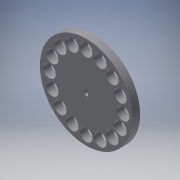
# Autodesk Inventor part: feeder_ring
Saved by Autodesk Inventor 2019 (Build 230136000, 136)
## iProperties
Created: 2018-11-14
Part Number: feeder_ring
Material: Generic
Document SubType Name: Modeling
Designer: chill
Density: 1 g/cm^3
Appearance: Default
Author: chill
Autodesk Inventor part; units mm, degrees
ref_plane "YZ Plane" through (0, 0, 0) normal (1, 0, 0) x (0, 1, 0)
ref_plane "XZ Plane" through (0, 0, 0) normal (0, 1, 0) x (-1, 0, 0)
ref_plane "XY Plane" through (0, 0, 0) normal (0, 0, 1) x (1, 0, 0)
sketch "Sketch1" plane through (0, 0, 0) normal (0, 0, 1) x (1, 0, 0)
  circle A0 centre (0, 29) radius 5
  circle A1 centre (0, 0) radius 36.5
  line L0 (-1.5, 2) -> (-1.5, 0)
  line L1 (-1.5, 0) -> (-1.5, -2)
  line L2 (1.5, 2) -> (1.5, 0)
  line L3 (1.5, 0) -> (1.5, -2)
  arc A2 (-1.5, -2) -> (1.5, -2) centre (0, 0) ccw
  arc A3 (1.5, 2) -> (-1.5, 2) centre (0, 0) ccw
  circle A4 centre (-11.0978, 26.7925) radius 5
  circle A5 centre (-20.5061, 20.5061) radius 5
  circle A6 centre (-26.7925, 11.0978) radius 5
  circle A7 centre (-29, 0) radius 5
  circle A8 centre (-26.7925, -11.0978) radius 5
  circle A9 centre (-20.5061, -20.5061) radius 5
  circle A10 centre (-11.0978, -26.7925) radius 5
  circle A11 centre (0, -29) radius 5
  circle A12 centre (11.0978, -26.7925) radius 5
  circle A13 centre (20.5061, -20.5061) radius 5
  circle A14 centre (26.7925, -11.0978) radius 5
  circle A15 centre (29, 0) radius 5
  circle A16 centre (26.7925, 11.0978) radius 5
  circle A17 centre (20.5061, 20.5061) radius 5
  circle A18 centre (11.0978, 26.7925) radius 5
  dimension "d15" = 29
  dimension "d18" = 360
  dimension "d20" = 10
  dimension "d21" = 73
  dimension "d35" = 2.5
  dimension "d36" = 2.5
  dimension "d37" = 3
  dimension "d38" = 1.5
  dimension "d39" = 1.5
  dimension "d40" = 1.5
  dimension "d41" = 27.5
  dimension "d42" = 27.5
  dimension "d43" = 28.2925
  dimension "d44" = 1.5
  dimension "d45" = 2.5
  constraints: 19 centre point, 8 end point, 4 point on circle, 1 coincident, 1 parallel, 1 vertical, 33 other
  measures "d15" distance of point (0, 0) A0.centre
  measures "d20" diameter of A15
  measures "d21" diameter of A1
  measures "d35" radius of A3
  measures "d36" radius of A2
  measures "d37" distance between parallel lines of L3 L1
  measures "d38" distance from line of point (0, 0) L2
  measures "d39" distance from line of point (0, 0) L3
  measures "d40" distance from line of point (0, 0) L0
  measures "d41" distance from line of A15.centre L2
  measures "d42" distance from line of A15.centre L3
  measures "d43" distance from line of A16.centre L0
  measures "d44" distance from line of A1.centre L2
  measures "d45" distance of point (0, 0) L2.start
extrude "Extrusion1" add sketch "Sketch1" along normal blind 6
body "Solid1"
